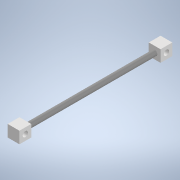
# Autodesk Inventor part: srodek
Saved by Autodesk Inventor 2021 (Build 250183000, 183)
## iProperties
Created: 2021-10-08
Part Number: srodek
Material: Generic
Document SubType Name: Modeling
Designer: nikod
Density: 1 g/cm^3
Appearance: Default
Author: nikod
Autodesk Inventor part; units mm, degrees
ref_plane "YZ Plane" through (0, 0, 0) normal (1, 0, 0) x (0, 1, 0)
ref_plane "XZ Plane" through (0, 0, 0) normal (0, 1, 0) x (-1, 0, 0)
ref_plane "XY Plane" through (0, 0, 0) normal (0, 0, 1) x (1, 0, 0)
sketch "Sketch1" plane through (0, 0, 0) normal (0, 0, 1) x (1, 0, 0)
  line L0 (1604.4809, 6805.3292) -> (1804.4809, 6805.3292)
  line L1 (1804.4809, 6805.3292) -> (1804.4809, 6605.3292)
  line L2 (1804.4809, 6605.3292) -> (1604.4809, 6605.3292)
  line L3 (1604.4809, 6605.3292) -> (1604.4809, 6805.3292)
  point P0 (0, 0)
  dimension "d0" = 200
  dimension "d1" = 200
  constraints: 8 end point, 2 parallel, 1 horizontal, 1 perpendicular
  measures "d0" distance of L1.end L2.end
  measures "d1" distance of L0.end L1.end
extrude "Extrusion1" add sketch "Sketch1" along normal blind 200
sketch "Sketch2" plane through (0, 0, 200) normal (0, 0, 1) x (1, 0, 0)
  line L0 (1804.4809, 6805.3292) -> (1604.4809, 6805.3292) projected
  line L1 (1604.4809, 6605.3292) -> (1804.4809, 6605.3292) projected
  circle A0 centre (1704.4809, 6705.3292) radius 45
  point P0 (0, 0)
  dimension "d4" = 90
  constraints: 1 centre point
  measures "d4" diameter of A0
extrude "Extrusion2" add sketch "Sketch2" along normal blind 1100
sketch "Sketch4" plane through (1804.4809, 6605.3292, 0) normal (1, 0, 0) x (0, 0, -1)
  line L0 (0, 200) -> (-200, 200) projected
  line L1 (-100, 200) -> (-100, 0)
  line L2 (0, 0) -> (-200, 0) projected
  circle A0 centre (-100, 100) radius 45
  point P0 (0, -6605.3292)
  dimension "d12" = 90
  constraints: 3 midpoint, 2 end point, 1 centre point
  measures "d12" diameter of A0
extrude "Extrusion4" cut sketch "Sketch4" against normal blind 200
mirror "Mirror1" about plane through (1704.4809, 6705.3292, 1300) normal (0, 0, 1) of "Extrusion2", "Extrusion1", "Extrusion4"
thread "Thread1" size "M90x6" class "6g" standard "ISO Metric profile" full length
body "Solid1"
